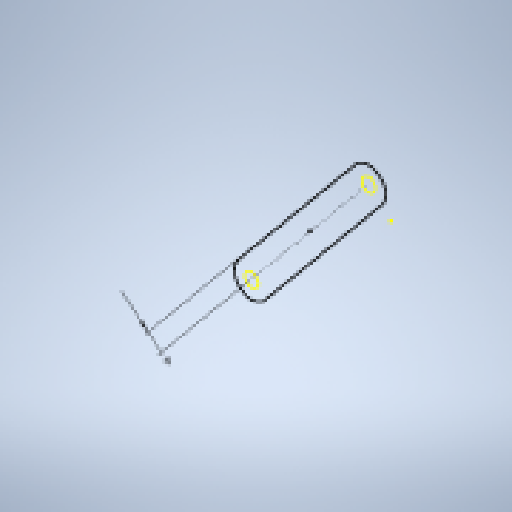
# Autodesk Inventor part: linkage-arm
Saved by Autodesk Inventor 2024.1 (Build 281209000, 209)
## iProperties
Created: 2025-06-12
Part Number: linkage-arm
Material: Generic
Document SubType Name: Modeling
Designer: iwheard
Density: 1 g/cm^3
Appearance: Default
Author: iwheard
Autodesk Inventor part; units mm, degrees
ref_plane "YZ Plane" through (0, 0, 0) normal (1, 0, 0) x (0, 1, 0)
ref_plane "XZ Plane" through (0, 0, 0) normal (0, 1, 0) x (-1, 0, 0)
ref_plane "XY Plane" through (0, 0, 0) normal (0, 0, 1) x (1, 0, 0)
sketch "Sketch1" plane through (0, 0, 0) normal (0, 0, 1) x (1, 0, 0)
  circle A0 centre (-5.1902, 4.697) radius 1.6 projected
  circle A1 centre (-32.4398, -28.1035) radius 1.6 projected
  line L0 (-32.4398, -28.1035) -> (-5.1902, 4.697) construction
  line L1 (-29.363, -30.6596) -> (-2.1134, 2.1409)
  line L2 (-8.267, 7.2531) -> (-35.5166, -25.5474)
  arc A2 (-35.5166, -25.5474) -> (-29.363, -30.6596) centre (-32.4398, -28.1035) ccw
  arc A3 (-2.1134, 2.1409) -> (-8.267, 7.2531) centre (-5.1902, 4.697) ccw
  point P0 (0, 0)
  point P1 (-18.815, -11.7033)
  dimension "d0" = 4
  constraints: 8 end point, 4 point on circle, 4 tangent, 2 centre point, 1 midpoint, 1 parallel
  measures "d0" distance between parallel lines of L2 L0
extrude "Extrusion1" add sketch "Sketch1" along normal blind 2
body "Solid1"
